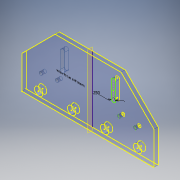
# Autodesk Inventor part: junk
Saved by Autodesk Inventor 2017 (Build 210142000, 142)
## iProperties
Created: 2017-05-17
Part Number: junk
Material: Water
Document SubType Name: Modeling
Designer: User
Density: 0.9983 g/cm^3
Appearance: Tropical Blue
Mass: 108.3 g
Surface Area: 399.87 cm^2
Volume: 108.484 cm^3
Author: User
Autodesk Inventor part; units mm, degrees
ref_plane "XZ Plane" through (0, 0, 0) normal (0, 1, 0) x (-1, 0, 0)
ref_plane "XY Plane" through (0, 0, 0) normal (0, 0, 1) x (1, 0, 0)
sketch "Sketch1" plane through (0, 0, 0) normal (0, 0, 1) x (1, 0, 0)
  line L0 (0, 0) -> (203.2, 0)
  line L1 (203.2, 0) -> (203.2, 50.8)
  line L2 (152.4, 101.6) -> (50.8, 101.6)
  line L3 (0, 50.8) -> (0, 0)
  line L4 (50.8, 101.6) -> (0, 50.8)
  line L5 (152.4, 101.6) -> (203.2, 50.8)
  point P0 (203.2, 101.6)
  point P1 (0, 101.6)
  dimension "d0" = 50.8
  dimension "d1" = 50.8
  dimension "d2" = 50.8
  dimension "d3" = 50.8
  dimension "d7" = 203.2
  dimension "d8" = 101.6
  constraints: 12 end point, 4 point on line, 2 parallel, 1 horizontal, 1 perpendicular
  measures "d0" distance of L2.end point (0, 101.6)
  measures "d1" distance of L3.start point (0, 101.6)
  measures "d2" distance of L2.start point (203.2, 101.6)
  measures "d3" distance of L1.end point (203.2, 101.6)
  measures "d7" distance of L0.start L0.end
  measures "d8" distance between parallel lines of L0 L2
extrude "Extrusion1" add sketch "Sketch1" along normal blind 6.35
sketch "Sketch2" plane through (0, 0, 6.35) normal (0, 0, 1) x (1, 0, 0)
  line L0 (0, 0) -> (203.2, 0) projected
  line L1 (0, 0) -> (203.2, 0) projected
  line L2 (203.2, 0) -> (203.2, 50.8) projected
  line L3 (203.2, 50.8) -> (152.4, 101.6) projected
  line L4 (152.4, 101.6) -> (50.8, 101.6) projected
  line L5 (50.8, 101.6) -> (0, 50.8) projected
  line L6 (0, 50.8) -> (0, 0) projected
  point P0 (25.4, 12.7)
  point P1 (76.1155, 12.7)
  dimension "d6" = 12.7
  dimension "d9" = 25.4
  measures "d6" distance from line of point (25.4, 12.7) L0
  measures "d9" distance from line of point (25.4, 12.7) L6
hole "Hole1" at (25.4, 12.7, 6.35) at (76.1155, 12.7, 6.35) direction (0, 0, -1) diameter 12.7 depth 25.4 tip angle 118
pattern_linear "Rectangular Pattern1" count 4 spacing 50.8 along (1, 0, 0) of "Hole1" first direction both ways yes
sketch "Sketch3" plane through (0, 0, 6.35) normal (0, 0, 1) x (1, 0, 0)
  line L0 (0, 0) -> (203.2, 0) projected
  line L1 (203.2, 0) -> (203.2, 50.8) projected
  line L2 (203.2, 50.8) -> (152.4, 101.6) projected
  line L3 (152.4, 101.6) -> (50.8, 101.6) projected
  line L4 (50.8, 101.6) -> (0, 50.8) projected
  line L5 (0, 50.8) -> (0, 0) projected
  arc A0 (76.1577, 6.3501) -> (76.1577, 19.0499) centre (76.2, 12.7) ccw projected
  arc A1 (76.1577, 19.0499) -> (76.1577, 6.3501) centre (76.1155, 12.7) ccw projected
  circle A2 centre (177.7155, 12.7) radius 6.35 projected
  arc A3 (126.9577, 6.3501) -> (126.9577, 19.0499) centre (127, 12.7) ccw projected
  arc A4 (126.9577, 19.0499) -> (126.9577, 6.3501) centre (126.9155, 12.7) ccw projected
  arc A5 (25.3577, 19.0499) -> (25.3577, 6.3501) centre (25.3155, 12.7) ccw projected
  arc A6 (25.3577, 6.3501) -> (25.3577, 19.0499) centre (25.4, 12.7) ccw projected
  line L6 (140.7734, 84.608) -> (140.7734, 58.6856) construction
  line L7 (152.4, 101.6) -> (50.8, 101.6) projected
  line L8 (137.5984, 84.608) -> (137.5984, 58.6856)
  line L9 (143.9484, 58.6856) -> (143.9484, 84.608)
  arc A7 (143.9484, 84.608) -> (137.5984, 84.608) centre (140.7734, 84.608) ccw
  arc A8 (137.5984, 58.6856) -> (143.9484, 58.6856) centre (140.7734, 58.6856) ccw
  point P0 (140.7734, 71.6468)
  point P1 (174.2566, 38.1636)
  point P2 (149.4142, 41.0439)
  dimension "d20" = 6.35
  constraints: 8 end point, 4 point on circle, 4 tangent, 2 centre point, 1 midpoint, 1 parallel, 1 perpendicular
  measures "d20" diameter of A8
hole "Hole2" at (174.2566, 38.1636, 6.35) at (149.4142, 41.0439, 6.35) direction (0, 0, -1) diameter 4.9784 depth 19.05 tip angle 118 thread size "1/4-20 UNC" class "2B" standard "ANSI Unified Screw Threads"
extrude "Extrusion2" cut sketch "Sketch3" against normal blind 6.35 contours A7 L9 A8 L8
sketch "Sketch4" plane through (0, 0, 0) normal (0, 0, -1) x (-1, 0, 0)
  arc A0 (-143.9484, 58.6856) -> (-137.5984, 58.6856) centre (-140.7734, 58.6856) ccw projected
  line L0 (-143.9484, 58.6856) -> (-143.9484, 84.608) projected
  arc A1 (-137.5984, 84.608) -> (-143.9484, 84.608) centre (-140.7734, 84.608) ccw projected
  line L1 (-137.5984, 84.608) -> (-137.5984, 58.6856) projected
  circle A2 centre (-174.2566, 38.1636) radius 2.4892 projected
  circle A3 centre (-149.4142, 41.0439) radius 2.4892 projected
  line L2 (0, 0) -> (-203.2, 0) projected
  line L3 (0, 50.8) -> (0, 0) projected
  line L4 (-50.8, 101.6) -> (0, 50.8) projected
  line L5 (-152.4, 101.6) -> (-50.8, 101.6) projected
  line L6 (-203.2, 50.8) -> (-152.4, 101.6) projected
  line L7 (-203.2, 0) -> (-203.2, 50.8) projected
  arc A4 (-25.3577, 6.3501) -> (-25.3577, 19.0499) centre (-25.3155, 12.7) ccw projected
  arc A5 (-25.3577, 19.0499) -> (-25.3577, 6.3501) centre (-25.4, 12.7) ccw projected
  circle A6 centre (-177.7155, 12.7) radius 6.35 projected
  arc A7 (-126.9577, 19.0499) -> (-126.9577, 6.3501) centre (-127, 12.7) ccw projected
  arc A8 (-126.9577, 6.3501) -> (-126.9577, 19.0499) centre (-126.9155, 12.7) ccw projected
  arc A9 (-76.1577, 19.0499) -> (-76.1577, 6.3501) centre (-76.2, 12.7) ccw projected
  arc A10 (-76.1577, 6.3501) -> (-76.1577, 19.0499) centre (-76.1155, 12.7) ccw projected
  line L8 (-152.4, 101.6) -> (-50.8, 101.6) projected
  line L9 (-101.6, 101.6) -> (-101.6, 0)
  line L10 (0, 0) -> (-203.2, 0) projected
  constraints: 2 end point, 2 midpoint
ref_plane "Work Plane1" through (101.6, 101.6, 0) normal (1, 0, 0) x (0, -1, 0)
mirror "Mirror1" about plane through (101.6, 101.6, 0) normal (1, 0, 0) of "Extrusion2", "Hole2"
mirror "Mirror2" about plane through (101.6, 101.6, 0) normal (1, 0, 0) of "Extrusion1", "Extrusion2", "Hole2", "Mirror1", "Hole1", "Rectangular Pattern1"
sketch "Sketch5" plane through (0, 0, 0) normal (0, 0, -1) x (-1, 0, 0)
  line L0 (-91.0569, 50.3137) -> (-46.6879, 50.3137) construction
  line L1 (-46.6879, 50.3137) -> (-46.6879, 47.0459) construction
  line L2 (-46.6879, 47.0459) -> (-91.0569, 47.0459) construction
  line L3 (-91.0569, 47.0459) -> (-91.0569, 50.3137) construction
  point P0 (0, 0)
  constraints: 2 other
equation "\"d1\" = d0"
equation "\"d3\" = d2"
body "Solid1"
